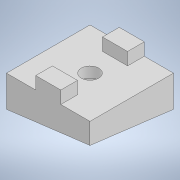
# Autodesk Inventor part: corner
Saved by Autodesk Inventor 2022 (Build 260153000, 153)
## iProperties
Created: 2021-10-04
Part Number: corner
Material: Generic
Document SubType Name: Modeling
Designer: tecware
Density: 1 g/cm^3
Appearance: Default
Author: tecware
## iProperties of the stored document corner_3DPrint.ipt
Created: 2021-10-04
Part Number: corner_3DPrint
Material: Generic
Document SubType Name: Modeling
Designer: tecware
Density: 1 g/cm^3
Appearance: Default
Author: tecware
Autodesk Inventor part; units mm, degrees
ref_plane "YZ Plane" through (0, 0, 0) normal (1, 0, 0) x (0, 1, 0)
sketch "Sketch1" plane through (0, 0, 0) normal (0, 1, 0) x (-1, 0, 0)
  line L0 (10, -10) -> (-10, -10)
  line L1 (-10, -10) -> (-10, 10)
  line L2 (-10, 10) -> (10, 10)
  line L3 (10, 10) -> (10, -10)
  dimension "d0" = 20
  dimension "d1" = 20
  constraints: 8 end point, 2 parallel, 1 horizontal, 1 perpendicular
  measures "d0" distance of L1.end L2.end
  measures "d1" distance of L0.end L1.end
extrude "Main Body Extrusion" add sketch "Sketch1" against normal blind 10
ref_plane "Work Plane1" through (10, 0, 10) normal (0.7071, 0, -0.7071) x (0, -1, 0)
sketch "Sketch2" plane through (10, 0, 10) normal (0.7071, 0, -0.7071) x (0, -1, 0)
  line L0 (0, 0) -> (10, 0) projected
  line L1 (10, 14.1421) -> (10, 28.2843) projected
  line L2 (5, 0) -> (10, 28.2843)
  line L3 (5, 0) -> (10, 0)
  line L4 (10, 0) -> (10, 14.1421) projected
  line L5 (10, 14.1421) -> (10, 0)
  point P0 (0, 14.1421)
  constraints: 6 end point, 1 collinear, 1 midpoint, 1 perpendicular
extrude "Slanted Cut" cut sketch "Sketch2" along normal through all both and the other way through all
sketch "Sketch3" plane through (0, 0, 0) normal (0, 1, 0) x (1, 0, 0)
  point P0 (0, 0)
  point P1 (0, 0)
  constraints: 1 coincident
hole "Screw Hole" at (0, 0, 0) direction (0, -1, 0) diameter 4.2 end through all
ref_plane "Work Plane2" through (0, -10, 0) normal (0, 1, 0) x (1, 0, 0)
sketch "Sketch4" plane through (0, -10, 0) normal (0, 1, 0) x (1, 0, 0)
  circle A0 centre (0, 0) radius 4
  dimension "d14" = 8
  constraints: 1 centre point, 1 coincident
  measures "d14" diameter of A0
extrude "Counterbore for Screw Hole" cut sketch "Sketch4" along normal blind 7.5
sketch "Sketch5" plane through (0, 0, 0) normal (0, 1, 0) x (1, 0, 0)
  line L0 (-10, -10) -> (10, -10) projected
  line L1 (3, -10) -> (-3, -10)
  line L2 (-3, -10) -> (-3, 10)
  line L3 (-3, 10) -> (3, 10)
  line L4 (3, 10) -> (3, -10)
  circle A0 centre (0, 0) radius 2.1 projected
  line L5 (3, 10) -> (-3, 10)
  line L6 (-3, 10) -> (-3, 6)
  line L7 (-3, 6) -> (3, 6)
  line L8 (3, 6) -> (3, 10)
  line L9 (3, -10) -> (-3, -10)
  line L10 (-3, -10) -> (-3, -6)
  line L11 (-3, -6) -> (3, -6)
  line L12 (3, -6) -> (3, -10)
  constraints: 24 end point, 6 parallel, 3 horizontal, 3 perpendicular, 3 point on line
extrude "Alignment Extrusion" add sketch "Sketch5" along normal blind 3 contours L2 L11 L4 L0 | L2 L3 L4 L7
body "Solid1"
